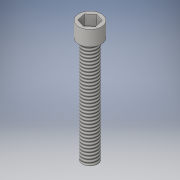
# Autodesk Inventor part: qtr20_75
Saved by Autodesk Inventor 2016 SP1 (Build 200210100, 210)
## iProperties
Created: 2015-12-11
Part Number: qtr20_75
Material: Generic
Document SubType Name: Modeling
Designer: ddeboer
Density: 1 g/cm^3
Appearance: Default
Author: ddeboer
Autodesk Inventor part; units mm, degrees
ref_plane "YZ Plane" through (0, 0, 0) normal (1, 0, 0) x (0, 1, 0)
ref_plane "XZ Plane" through (0, 0, 0) normal (0, 1, 0) x (-1, 0, 0)
ref_plane "XY Plane" through (0, 0, 0) normal (0, 0, 1) x (1, 0, 0)
sketch "Sketch1" plane through (0, 0, 0) normal (0, 1, 0) x (-1, 0, 0)
  circle A0 centre (0, 0) radius 3.175
  dimension "d2" = 6.35
  constraints: 1 centre point, 1 coincident
  measures "d2" diameter of A0
extrude "Extrusion1" add sketch "Sketch1" along normal blind 44.45
thread "Thread1" size "1/4-20 UNC" class "2A" standard "ANSI Unified Screw Threads" full length
sketch "Sketch2" plane through (0, 44.45, 0) normal (0, 1, 0) x (1, 0, 0)
  circle A0 centre (0, 0) radius 4.7625
  dimension "d7" = 9.525
  constraints: 1 centre point, 1 coincident
  measures "d7" diameter of A0
extrude "Extrusion2" add sketch "Sketch2" along normal blind 6.35
sketch "Sketch3" plane through (0, 50.8, 0) normal (0, 1, 0) x (1, 0, 0)
  line L0 (2.719, 2.4592) -> (3.4893, -1.1251)
  line L1 (3.4893, -1.1251) -> (0.7703, -3.5843)
  line L2 (0.7703, -3.5843) -> (-2.719, -2.4592)
  line L3 (-2.719, -2.4592) -> (-3.4893, 1.1251)
  line L4 (-3.4893, 1.1251) -> (-0.7703, 3.5843)
  line L5 (-0.7703, 3.5843) -> (2.719, 2.4592)
  point P0 (0, 0)
  point P1 (0, 0)
  dimension "d10" = 6.35
  constraints: 12 end point, 1 coincident, 13 other
  measures "d10" distance between parallel lines of L3 L0
extrude "Extrusion3" cut sketch "Sketch3" against normal blind 4.318
body "Solid1"
